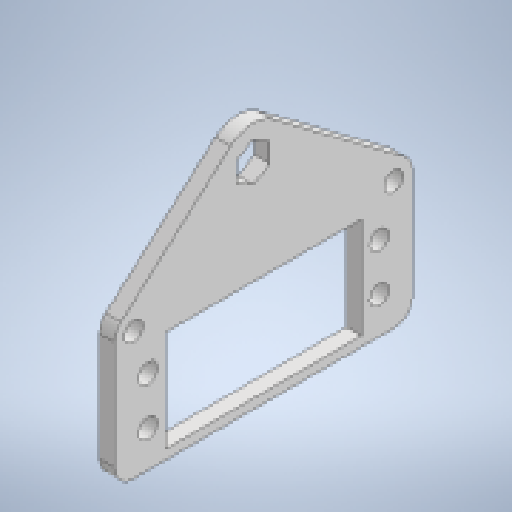
# Autodesk Inventor part: servoPlate
Saved by Autodesk Inventor 2023 (Build 270158000, 158)
## iProperties
Created: 2022-09-10
Part Number: servoPlate
Material: Generic
Document SubType Name: Modeling
Designer: deli
Density: 1 g/cm^3
Appearance: Default
Author: deli
Autodesk Inventor part; units mm, degrees
ref_plane "YZ Plane" through (0, 0, 0) normal (1, 0, 0) x (0, 1, 0)
ref_plane "XZ Plane" through (0, 0, 0) normal (0, 1, 0) x (-1, 0, 0)
ref_plane "XY Plane" through (0, 0, 0) normal (0, 0, 1) x (1, 0, 0)
sketch "Sketch1" plane through (0, 0, 0) normal (1, 0, 0) x (0, 1, 0)
  circle A0 centre (108.0055, 245.517) radius 2
  circle A1 centre (108.0055, 197.517) radius 2
  circle A2 centre (98.1055, 197.517) radius 2
  circle A3 centre (98.1055, 245.517) radius 2
  line L0 (108.0055, 245.517) -> (108.0055, 197.517) construction
  line L1 (108.0055, 197.517) -> (98.1055, 197.517) construction
  line L2 (98.1055, 197.517) -> (98.1055, 245.517) construction
  line L3 (98.1055, 245.517) -> (108.0055, 245.517) construction
  line L4 (113.0555, 248.667) -> (93.0555, 248.667) construction
  line L5 (93.0555, 248.667) -> (93.0555, 194.367) construction
  line L6 (93.0555, 194.367) -> (113.0555, 194.367) construction
  line L7 (113.0555, 194.367) -> (113.0555, 248.667) construction
  line L8 (113.0555, 241.367) -> (93.0555, 241.367) construction
  line L9 (93.0555, 241.367) -> (93.0555, 201.667) construction
  line L10 (93.0555, 201.667) -> (113.0555, 201.667) construction
  line L11 (113.0555, 201.667) -> (113.0555, 241.367) construction
  line L12 (92.5555, 241.867) -> (113.5555, 241.867)
  line L13 (113.5555, 241.867) -> (113.5555, 201.167)
  line L14 (113.5555, 201.167) -> (92.5555, 201.167)
  line L15 (92.5555, 201.167) -> (92.5555, 241.867)
  circle A4 centre (117.0555, 248.517) radius 2
  circle A5 centre (117.0555, 194.517) radius 2
  arc A6 (120.0472, 251.1722) -> (117.0555, 252.517) centre (117.0555, 248.517) ccw
  arc A7 (117.0555, 190.517) -> (120.2639, 192.1282) centre (117.0555, 194.517) ccw
  arc A8 (90.5555, 194.517) -> (94.5555, 190.517) centre (94.5555, 194.517) ccw
  arc A9 (94.5555, 252.517) -> (90.5555, 248.517) centre (94.5555, 248.517) ccw
  line L16 (121.0555, 248.1479) -> (121.0555, 194.1479) construction
  line L17 (117.0555, 190.517) -> (94.5555, 190.517)
  line L18 (90.5555, 194.517) -> (90.5555, 248.517)
  line L19 (94.5555, 252.517) -> (117.0555, 252.517)
  line L20 (131.0141, 223.717) -> (133.0348, 227.217)
  line L21 (133.0348, 227.217) -> (137.0762, 227.217)
  line L22 (137.0762, 227.217) -> (139.097, 223.717)
  line L23 (139.097, 223.717) -> (137.0762, 220.217)
  line L24 (137.0762, 220.217) -> (133.0348, 220.217)
  line L25 (133.0348, 220.217) -> (131.0141, 223.717)
  circle A10 centre (135.0555, 223.717) radius 7
  line L26 (120.0472, 251.1722) -> (140.2909, 228.3636)
  line L27 (140.6702, 219.5367) -> (120.2639, 192.1282)
  point P0 (0, 0)
  dimension "d0" = 4
  dimension "d1" = 4
  dimension "d2" = 4
  dimension "d3" = 4
  dimension "d4" = 9.9
  dimension "d5" = 48
  dimension "d7" = 20
  dimension "d8" = 5.05
  dimension "d9" = 3.15
  dimension "d10" = 39.7
  dimension "d11" = 7.3
  dimension "d12" = 0.5
  dimension "d14" = 4
  dimension "d16" = 4
  dimension "d18" = 2
  dimension "d20" = 2
  dimension "d28" = 54
  dimension "d30" = 2
  dimension "d31" = 7.5
  dimension "d32" = 62
  dimension "d33" = 3.85
  dimension "d34" = 54.3
  dimension "d35" = 7
  dimension "d36" = 14
  dimension "d37" = 14
  dimension "d40" = 54
  dimension "d41" = 26.2
  constraints: 56 end point, 12 tangent, 11 centre point, 10 point on circle, 9 perpendicular, 6 parallel, 3 coincident, 3 horizontal, 2 point on line, 2 vertical, 16 other
  measures "d0" diameter of A0
  measures "d1" diameter of A3
  measures "d2" diameter of A1
  measures "d3" diameter of A2
  measures "d4" distance of L2.end L0.start
  measures "d5" distance of L0.start L0.end
  measures "d7" distance of L5.end L6.end
  measures "d8" distance between parallel lines of L0 L7
  measures "d9" distance between parallel lines of L6 L1
  measures "d10" distance of L10.end L8.start
  measures "d11" distance between parallel lines of L6 L10
  measures "d12" distance between parallel lines of L8 L12
  measures "d14" diameter of A4
  measures "d16" diameter of A5
  measures "d18" radial gap between concentric circles of A6 A4
  measures "d20" radial gap between concentric circles of A5 A7
  measures "d28" distance of L16.start L16.end
  measures "d30" distance between parallel lines of L15 L18
  measures "d31" distance between parallel lines of L16 L13
  measures "d32" distance between parallel lines of L17 L19
  measures "d33" distance between parallel lines of L19 L4
  measures "d34" distance of L6.end L4.start
  measures "d35" distance between parallel lines of L24 L21
  measures "d36" diameter of A10
  measures "d37" distance from line of L16 point (135.056, 223.717)
  measures "d40" distance of A5.centre A4.centre
  measures "d41" vertical distance of L0.end A10.centre
extrude "Extrusion2" add sketch "Sketch1" along normal blind 3.175
equation "\"d1\" = d0"
equation "\"d2\" = d0"
equation "\"d3\" = d0"
equation "\"d8\" = -0.5 * d4 + 0.5 * d7"
equation "\"d9\" = -0.5 * d5 + 0.5 * d6"
equation "\"d11\" = -0.5 * d10 + 0.5 * d6"
equation "\"d14\" = d13"
equation "\"d16\" = d13"
equation "\"d18\" = d17"
equation "\"d20\" = d17"
equation "\"d33\" = -0.5 * d34 + 0.5 * d32"
equation "\"d40\" = d28"
equation "\"d6\" = 54.3"
equation "\"d13\" = 4"
equation "\"d17\" = 2"
body "Solid2"
